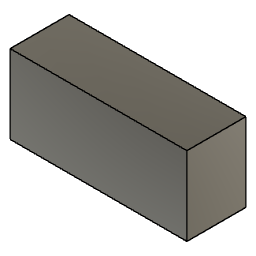
test v1 (Autodesk Fusion 360 design; units mm, degrees)
Autodesk Fusion 360 part; units mm, degrees
sketch "Sketch1" plane through (0, 0, 0) normal (0, 1, 0) x (1, 0, 0)
  line L0 (-60, -45) -> (30, -45)
  line L1 (30, -45) -> (30, -5)
  line L2 (30, -5) -> (-60, -5)
  line L3 (-60, -5) -> (-60, -45)
  constraint horizontal L0
  constraint vertical L1
  constraint horizontal L2
  constraint vertical L3
extrude "Extrude1" add sketch "Sketch1" along normal blind 30
